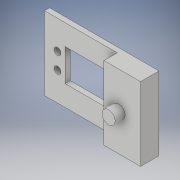
# Autodesk Inventor part: ClawServoHolder
Saved by Autodesk Inventor 2017 (Build 210142000, 142)
## iProperties
Created: 2017-09-23
Part Number: ClawServoHolder
Material: Generic
Document SubType Name: Modeling
Designer: User
Density: 1 g/cm^3
Appearance: Default
Author: User
Autodesk Inventor part; units mm, degrees
ref_plane "YZ Plane" through (0, 0, 0) normal (1, 0, 0) x (0, 1, 0)
ref_plane "XZ Plane" through (0, 0, 0) normal (0, 1, 0) x (-1, 0, 0)
ref_plane "XY Plane" through (0, 0, 0) normal (0, 0, 1) x (1, 0, 0)
sketch "Sketch1" plane through (0, 0, 0) normal (0, 0, 1) x (1, 0, 0)
  line L0 (0, 0) -> (38.8112, 0)
  line L1 (38.8112, 0) -> (38.8112, 19.812)
  line L2 (38.8112, 19.812) -> (0, 19.812)
  line L3 (0, 19.812) -> (0, 0)
  line L4 (-12.7, -12.7) -> (-12.7, 32.512)
  line L5 (-12.7, 32.512) -> (51.5112, 32.512)
  line L6 (51.5112, 32.512) -> (51.5112, -12.7)
  line L7 (-12.7, -12.7) -> (51.5112, -12.7)
  dimension "d0" = 38.8112
  dimension "d1" = 19.812
  constraints: 16 end point, 3 perpendicular, 2 horizontal, 2 parallel
  measures "d0" distance of L2.end L1.end
  measures "d1" distance of L1.end L0.end
extrude "Extrusion1" add sketch "Sketch1" along normal blind 3.175
sketch "Sketch2" plane through (0, 0, 3.175) normal (0, 0, 1) x (1, 0, 0)
  line L0 (0, 19.812) -> (0, 0) projected
  circle A0 centre (-4.5974, 4.9022) radius 1.0541
  line L1 (38.8112, 19.812) -> (38.8112, 0) projected
  circle A1 centre (43.4086, 4.9022) radius 1.0541
  circle A2 centre (43.4086, 14.9098) radius 1.0541
  circle A3 centre (-4.5974, 14.9098) radius 1.0541
  circle A4 centre (-4.5974, 4.9022) radius 2.1082
  circle A5 centre (-4.5974, 14.9098) radius 2.1082
  circle A6 centre (43.4086, 14.9098) radius 2.1082
  circle A7 centre (43.4086, 4.9022) radius 2.1082
  dimension "d10" = 2.1082
  dimension "d15" = 4.2164
  dimension "d16" = 4.2164
  dimension "d17" = 4.2164
  dimension "d18" = 4.2164
  constraints: 8 centre point, 5 coincident
  measures "d10" diameter of A0
  measures "d15" diameter of A4
  measures "d16" diameter of A5
  measures "d17" diameter of A6
  measures "d18" diameter of A7
extrude "Extrusion2" cut sketch "Sketch2" against normal blind 3.175 contours A0 | A1 | A2 | A3 | A4 | A5 | A6 | A7
sketch "Sketch3" plane through (51.5112, -12.7, 0) normal (1, 0, 0) x (0, 0, -1)
  line L0 (0, 0) -> (-3.175, 0) projected
  line L1 (-3.175, 0) -> (-3.175, 45.212) projected
  line L2 (0, 0) -> (-3.175, 0)
  line L3 (-3.175, 0) -> (-3.175, 45.212)
  line L4 (-3.175, 45.212) -> (0, 45.212)
  line L5 (0, 45.212) -> (0, 0)
  point P0 (0, 12.7)
  constraints: 8 end point, 2 parallel, 1 horizontal, 1 perpendicular
extrude "Extrusion3" add sketch "Sketch3" along normal blind 3.175
sketch "Sketch4" plane through (0, 0, 3.175) normal (0, 0, 1) x (1, 0, 0)
  line L0 (54.6862, 32.512) -> (54.6862, -12.7) projected
  line L1 (54.6862, 32.512) -> (51.5112, 32.512)
  line L2 (-12.7, 32.512) -> (54.6862, 32.512) projected
  line L3 (51.5112, 32.512) -> (51.2299, -12.7)
  line L4 (-12.7, -12.7) -> (54.6862, -12.7) projected
  line L5 (54.6862, -12.7) -> (51.2299, -12.7)
  point P0 (0, 0)
  dimension "d21" = 3.175
  constraints: 6 end point, 2 point on line, 1 collinear
  measures "d21" distance of L0.start L1.end
extrude "Extrusion4" add sketch "Sketch4" along normal blind 8.2296
sketch "Sketch8" plane through (0, 0, 3.175) normal (0, 0, 1) x (1, 0, 0)
  line L0 (51.2299, -12.7) -> (32.1799, -12.7)
  line L1 (-12.7, -12.7) -> (51.2299, -12.7) projected
  line L2 (38.8112, 0) -> (0, 0) projected
  line L3 (32.1799, -12.7) -> (32.1799, 32.512)
  line L4 (-12.7, 32.512) -> (51.5112, 32.512) projected
  line L5 (32.1799, 32.512) -> (51.5112, 32.512)
  line L6 (51.2299, -12.7) -> (51.5112, 32.512) projected
  line L7 (51.5112, 32.512) -> (51.2299, -12.7)
  dimension "d33" = 19.05
  dimension "d36" = 45.212
  constraints: 8 end point, 2 collinear, 2 point on line
  measures "d33" distance of L0.start L0.end
  measures "d36" distance of L0.end L3.end
extrude "Extrusion7" add sketch "Sketch8" along normal blind 8.2296
sketch "Sketch9" plane through (0, 0, 11.4046) normal (0, 0, 1) x (1, 0, 0)
  line L0 (54.6862, -12.7) -> (54.6862, 32.512) projected
  line L1 (54.6862, 8.6893) -> (68.1482, 8.6893) construction
  line L2 (-12.7, 32.512) -> (54.6862, 32.512) projected
  line L3 (41.2242, 32.512) -> (63.8302, 32.512) construction
  circle A0 centre (41.2242, 9.906) radius 4.0005
  point P0 (0, 0)
  dimension "d41" = 8.001
  constraints: 4 end point, 2 horizontal, 2 point on line, 1 centre point
  measures "d41" diameter of A0
extrude "Extrusion8" add sketch "Sketch9" along normal blind 6.1976
sketch "Sketch10" plane through (0, 0, 3.175) normal (0, 0, -1) x (-1, 0, 0)
  line L0 (-38.8112, 0) -> (-38.8112, 19.812) projected
  line L1 (-38.8112, 19.812) -> (-38.8112, 0)
  line L2 (-38.8112, 0) -> (-32.1799, 0)
  line L3 (-32.1799, 32.512) -> (-32.1799, -12.7) projected
  line L4 (-32.1799, 19.812) -> (-32.1799, 0)
  line L5 (-38.8112, 19.812) -> (0, 19.812) projected
  line L6 (-38.8112, 19.812) -> (-32.1799, 19.812)
  point P0 (0, 0)
  constraints: 8 end point, 3 collinear, 2 point on line, 1 perpendicular
extrude "Extrusion9" cut sketch "Sketch10" against normal blind 5.08
body "Solid1"
